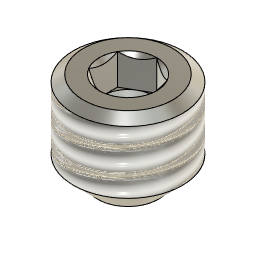
OH2A7A1-500 - SARI (Autodesk Fusion 360 archive; units mm, degrees)
design "92311A102 - SET SCREW, 4-40 X .093 CUP POINT, 18-8"
description: SET SCREW, 4-40 X .093 CUP POINT, 18-8
part number: 92311A102
Autodesk Fusion 360 part; units mm, degrees
sketch "Sketch1" plane through (0, 0, 0) normal (0, 0, 1) x (1, 0, 0)
  circle A0 centre (0, 0) radius 1.4224
  dimension "d7" = 2.8448
  constraint coincident A0.centre origin
  measures "d7" diameter of A0
extrude "Extrude1" add sketch "Sketch1" against normal blind 2.3813
sketch "Sketch2" plane through (0, 0, 0) normal (0, 0, 1) x (-1, 0, 0)
  circle A0 centre (0, 0) radius 1.4224
  line L0 (-0.635, -0.3666) -> (0, -0.7332)
  line L1 (0, -0.7332) -> (0.635, -0.3666)
  line L2 (0.635, -0.3666) -> (0.635, 0.3666)
  line L3 (0.635, 0.3666) -> (0, 0.7332)
  line L4 (0, 0.7332) -> (-0.635, 0.3666)
  line L5 (-0.635, 0.3666) -> (-0.635, -0.3666)
  dimension "d10" = 1.27
  constraint coincident A0.centre origin
  constraint vertical L5
  measures "d10" distance of L1.end L5
extrude "Extrude2" cut sketch "Sketch2" against normal blind 0.7874 contours L0 L1 L2 L3 L4 L5
sketch "Sketch3" plane through (0, 0, 0) normal (0, 1, 0) x (1, 0, 0)
  line L0 (1.4224, 0) -> (1.4224, 2.3813) construction
  line L1 (-1.4224, 2.3813) -> (-1.4224, 0) construction
  line L2 (-1.4224, 0) -> (-0.635, 0) construction
  line L3 (0.635, 0) -> (1.4224, 0) construction
  line L4 (1.4224, 2.3813) -> (-1.4224, 2.3813) construction
  line L5 (0, 0) -> (0, 2.3813)
  line L6 (0, 1.9158) -> (0.7747, 2.3813)
  line L7 (0.7747, 2.3813) -> (1.4224, 1.7335)
  line L8 (1.143, 0) -> (1.4224, 0.1956)
  line L9 (1.4224, 0.1956) -> (1.4224, 0)
  line L10 (1.4224, 0) -> (1.143, 0)
  line L11 (0, 1.9158) -> (-0.7747, 2.3813)
  line L12 (-0.7747, 2.3813) -> (-1.4224, 1.7335)
  line L13 (0, 2.3813) -> (0.7747, 2.3813)
  line L14 (0.7747, 2.3813) -> (1.4224, 2.3813)
  line L15 (1.4224, 2.3813) -> (1.4224, 1.7335)
  line L16 (-0.635, 0.7874) -> (0.635, 0.7874)
  line L17 (-0.635, 0.7874) -> (0, 1.154)
  line L18 (0, 1.154) -> (0.635, 0.7874)
  dimension "d13" = 35
  dimension "d14" = 45
  dimension "d15" = 118
  dimension "d16" = 1.5494
  dimension "d17" = 2.286
  dimension "d18" = 120
  constraint coincident L5.start origin
  constraint vertical L5
  constraint coincident L4 L5.end
  constraint coincident L5 L6.start
  constraint coincident L4 L6.end
  constraint coincident L0 L7.end
  constraint coincident L3 L8.start
  constraint coincident L0 L8.end
  constraint coincident L0.start L3.end
  constraint symmetric L5 L6.start L11.start
  constraint symmetric L5 L6.end L11.end
  constraint symmetric L5 L7.end L12.end
  constraint coincident L0.end L4.start
  constraint coincident L16.start L17.start
  constraint coincident L5 L17.end
  constraint coincident L16.end L18.end
  measures "d13" angle of L8 L10
  measures "d14" angle of L4 L7
  measures "d15" angle of L6 L11
  measures "d16" distance of L6.end L11.end
  measures "d18" angle of L17 L18
thread "Thread1" "ANSI Unified Screw Threads 0.112(#4) 4-40 UNC 3A" major diameter 2.7813 minor diameter 2.0879 pitch 0.635 angle 60 resizes the face on face at (1.4206, -0.0709, -1.5875)
revolve "Revolve1" cut sketch "Sketch3" angle 360 about axis through (0, 0, 0) along (0, 0, -1) contours L7 L14 L15 | L5 L6 L13 | L5 L16 L18 | L8 L9 L10
sketch "Sketch4" plane through (0, 0, 0) normal (1, 0, 0) x (0, 1, 0)
  line L0 (-0.7332, 0) -> (0.7332, 0)
  line L1 (0.7332, 0) -> (0, -0.7332)
  line L2 (0, -0.7332) -> (0, 0)
  line L3 (0, -0.7332) -> (-0.7332, 0)
  point P0 (0.7332, 0)
  point P1 (-0.7332, 0)
  dimension "d20" = 45
  constraint coincident P1 L0.start
  constraint coincident P0 L0.end
  constraint coincident L2.end origin
  constraint perpendicular L0 L2
  measures "d20" angle of L0 L3
revolve "Revolve2" cut sketch "Sketch4" angle 360 about axis through (0, 0, -0.7332) along (0, 0, 1) contours L0 L2 L3
equation "Length = ( 3 / 32 ) * 1 in" comment "Screw length"
equation "MajorDia = 0.112 in" comment "Thread major diameter"
equation "HexWidth = 0.05 in" comment "Hex drive socket width"
equation "CupDia = 0.061 in" comment "Cup diameter"
equation "MinorDia = 0.09 in" comment "Minor or top-face diameter"
equation "HexDepth = 0.031 in" comment "Hex socket depth"
equation "d7 = MajorDia"
equation "d8 = -Length"
equation "d10 = HexWidth"
equation "d11 = -HexDepth"
equation "d16 = CupDia"
equation "d17 = MinorDia"

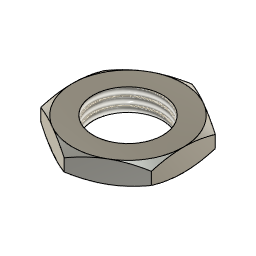
design "PEC11R NUT - HEX NUT FOR SWITCH, M7 X .75"
description: HEX NUT FOR SWITCH, M7 X .75
part number: PEC11R NUT
Autodesk Fusion 360 part; units mm, degrees
sketch "Sketch1" plane through (0, 0, 0) normal (0, 0, 1) x (1, 0, 0)
  line L0 (5, 2.8868) -> (0, 5.7735)
  line L1 (0, 5.7735) -> (-5, 2.8868)
  line L2 (-5, 2.8868) -> (-5, -2.8868)
  line L3 (-5, -2.8868) -> (0, -5.7735)
  line L4 (0, -5.7735) -> (5, -2.8868)
  line L5 (5, -2.8868) -> (5, 2.8868)
  circle A0 centre (0, 0) radius 5 construction
  dimension "d1" = 10
  constraint coincident A0.centre origin
  constraint vertical L5
  constraint tangent L5 A0
  measures "d1" distance of L2 L5
extrude "Extrude1" add sketch "Sketch1" along normal blind 2
sketch "Sketch2" plane through (0, 0, 0) normal (1, 0, 0) x (0, 1, 0)
  line L0 (5.7735, 2) -> (-5.7735, 2) construction
  line L1 (-5.7735, 0) -> (5.7735, 0) construction
  line L2 (-5, 0) -> (-5, 2) construction
  line L3 (0, 0) -> (0, 2)
  line L4 (-5.7735, 2) -> (-5.7735, 1.5534)
  line L5 (-5.7735, 1.5534) -> (-5, 2)
  line L6 (-5.7735, 2) -> (-5, 2)
  line L7 (-5.7735, 0) -> (-5.7735, 0.4466)
  line L8 (-5.7735, 0.4466) -> (-5, 0)
  line L9 (-5, 0) -> (-5.7735, 0)
  point P0 (-5, 0)
  point P1 (5, 0)
  dimension "d4" = 30
  constraint coincident P0 L2.start
  constraint coincident L0 L2.end
  constraint perpendicular L0 L2
  constraint coincident L3.start origin
  constraint midpoint L0 L3.end
  constraint coincident L0.end L4.start
  constraint perpendicular L0 L4
  constraint coincident L1.start L7.start
  constraint perpendicular L1 L7
  constraint equal L4 L7
  measures "d4" angle of L5 L6
revolve "Revolve1" cut sketch "Sketch2" angle 360 about axis through (0, 0, 0) along (0, 0, 1)
sketch "Sketch3" plane through (0, 0, 2) normal (0, 0, 1) x (-1, 0, 0)
  arc A0 (-2.5, -4.3301) -> (2.5, -4.3301) centre (0, 0) ccw
  arc A1 (2.5, -4.3301) -> (5, 0) centre (0, 0) ccw
  arc A2 (5, 0) -> (2.5, 4.3301) centre (0, 0) ccw
  arc A3 (2.5, 4.3301) -> (-2.5, 4.3301) centre (0, 0) ccw
  arc A4 (-2.5, 4.3301) -> (-5, 0) centre (0, 0) ccw
  arc A5 (-5, 0) -> (-2.5, -4.3301) centre (0, 0) ccw
  constraint coincident A0.centre A1.centre
hole "Hole1" at (0, 0, 2) direction (0, 0, -1) diameter 6.283 end through all
thread "Thread1" "ISO Metric profile 7.0 M7x0.75 6H"

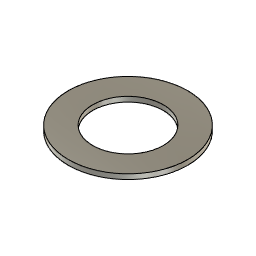
design "PEC11R WASHER - WASHER FOR SWITCH, M7, 12 MM OD"
description: WASHER FOR SWITCH, M7, 12 MM OD
part number: PEC11R WASHER
Autodesk Fusion 360 part; units mm, degrees
sketch "Sketch1" plane through (0, 0, 0) normal (0, 0, 1) x (1, 0, 0)
  circle A0 centre (0, 0) radius 6
  circle A1 centre (0, 0) radius 3.55
  dimension "d1" = 12
  dimension "d2" = 7.1
  constraint coincident A0.centre A1.centre
  constraint concentric A0 A1
  measures "d1" diameter of A0
  measures "d2" diameter of A1
extrude "Extrude1" add sketch "Sketch1" along normal blind 0.5
